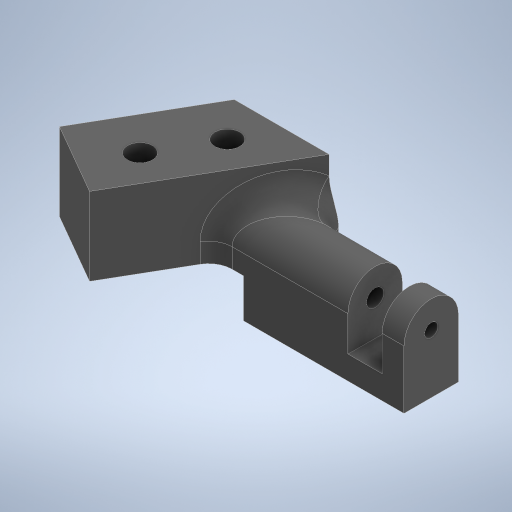
# Autodesk Inventor part: chain_base_connector
Saved by Autodesk Inventor 2024.1 (Build 281209000, 209)
## iProperties
Created: 2025-01-18
Part Number: chain_base_connector
Material: 一般
Document SubType Name: Modeling
Designer: hibik
Density: 1 g/cm^3
Appearance: 既定
Author: hibik
Autodesk Inventor part; units mm, degrees
ref_plane "YZ Plane" through (0, 0, 0) normal (1, 0, 0) x (0, 1, 0)
ref_plane "XZ Plane" through (0, 0, 0) normal (0, 1, 0) x (-1, 0, 0)
ref_plane "XY Plane" through (0, 0, 0) normal (0, 0, 1) x (1, 0, 0)
sketch "スケッチ1" plane through (0, 0, 0) normal (0, 1, 0) x (-1, 0, 0)
  line L0 (0, 0) -> (0, -18) construction
  line L1 (10, 0) -> (10, -23.7735) construction
  line L2 (10, -23.7735) -> (1.7863, -38)
  line L3 (10, -23.7735) -> (0, -18)
  line L4 (1.7863, -38) -> (-11.547, -38)
  line L5 (0, -18) -> (-11.547, -38) construction
  line L6 (-10.3923, -38) -> (0.866, -18.5)
  line L7 (9.5, -24.6395) -> (-0.9082, -18.6303)
  line L8 (-19, -38) -> (-29, -38)
  line L9 (-29, -38) -> (-29, 0)
  line L10 (-29, 0) -> (-19, 0)
  line L11 (-19, 0) -> (-19, -38)
  line L12 (-30, -38) -> (-30, 0.0797)
  line L13 (-5.1962, -36) -> (-29, -36)
  line L14 (-29, -36) -> (-29, -29)
  line L15 (-29, -29) -> (-5.1962, -29)
  line L16 (-5.1962, -29) -> (-5.1962, -36)
  point P0 (0.366, -19.366)
  point P1 (-9.2376, -36)
  dimension "d0" = 18
  dimension "d1" = 10
  dimension "d2" = 60
  dimension "d3" = 38
  dimension "d4" = 1
  dimension "d5" = 1
  dimension "d8" = 40
  dimension "d9" = 1
  dimension "d10" = 10
  dimension "d11" = 2
  dimension "d12" = 7
  constraints: 34 end point, 6 point on line, 5 parallel, 5 perpendicular, 3 horizontal, 3 vertical, 2 collinear
  measures "d0" distance of L0.start L0.end
  measures "d1" distance between parallel lines of L1 L0
  measures "d2" angle of L0 L3
  measures "d3" distance from line of L0.start L4
  measures "d4" distance between parallel lines of L5 L6
  measures "d5" distance between parallel lines of L3 L7
  measures "d8" distance from line of L1.start L12
  measures "d9" distance between parallel lines of L12 L9
  measures "d10" distance of L8.start L8.end
  measures "d11" distance between parallel lines of L8 L13
  measures "d12" distance of L15.end L13.start
extrude "押し出し1" add sketch "スケッチ1" along normal blind 3 contours L2 L7 L6 L3 | L2 L4 L6 L13 L16 L7 | L16 L13 L6 | L6 L13 L11 L15 | L11 L13 L9 L15
extrude "押し出し2" add sketch "スケッチ1" along normal blind 15 contours L2 L7 L6 L3 | L2 L4 L6 L13 L16 L7 | L16 L13 L6
sketch "スケッチ2" plane through (29, 0, -29) normal (1, 0, 0) x (0, 0, -1)
  circle A0 centre (3.5, 7.5) radius 0.85
  circle A1 centre (3.5, 7.5) radius 3.5
  line L0 (0, 7.5) -> (7, 7.5)
  line L1 (7, 7.5) -> (7, 3)
  line L2 (7, 3) -> (0, 3)
  line L3 (0, 3) -> (0, 7.5)
  line L4 (0, 3) -> (7, 3) projected
  line L5 (0, 0) -> (0, 3) projected
  point P0 (-29, 0)
  dimension "d16" = 7
  dimension "d15" = 1.7
  dimension "d17" = 4.5
  constraints: 8 end point, 2 collinear, 2 parallel, 2 vertical, 1 centre point, 1 coincident, 1 horizontal, 1 perpendicular, 3 other
  measures "d15" diameter of A0
  measures "d17" distance between parallel lines of L0 L2
extrude "押し出し3" add sketch "スケッチ2" against normal blind 2.8 contours L0 A1 A0 | A0 L0 A1 | L1 L2 L3 A1
ref_plane "作業平面1" through (24, 0, -29) normal (1, 0, 0) x (0, 0, -1)
mirror "ミラー1" about plane through (24, 0, -29) normal (1, 0, 0) of "押し出し3"
sketch "スケッチ3" plane through (19, 3, -29) normal (-1, 0, 0) x (0, 0, 1)
  circle A0 centre (-3.5, 4.5) radius 0.85 projected
  circle A1 centre (-3.5, 4.5) radius 1.1
  point P0 (29, -3)
  dimension "d21" = 2.2
  constraints: 1 centre point, 1 coincident
  measures "d21" diameter of A1
extrude "押し出し4" cut sketch "スケッチ3" against normal up to surface (2.8 mm away) contours A0 | A1
sketch "スケッチ5" plane through (0, 0, 0) normal (0, -1, 0) x (1, 0, 0)
  line L0 (3.814, -30.3) -> (5.4594, -33.15)
  line L1 (5.4594, -33.15) -> (3.814, -36)
  line L2 (3.814, -36) -> (0.5231, -36)
  line L3 (0.5231, -36) -> (-1.1224, -33.15)
  line L4 (-1.1224, -33.15) -> (0.5231, -30.3)
  line L5 (0.5231, -30.3) -> (3.814, -30.3)
  line L6 (-5.2246, -26.0447) -> (-3.5792, -23.1947)
  line L7 (-3.5792, -23.1947) -> (-0.2883, -23.1947)
  line L8 (-0.2883, -23.1947) -> (1.3571, -26.0447)
  line L9 (1.3571, -26.0447) -> (-0.2883, -28.8947)
  line L10 (-0.2883, -28.8947) -> (-3.5792, -28.8947)
  line L11 (-3.5792, -28.8947) -> (-5.2246, -26.0447)
  line L12 (-1.7863, -38) -> (-10, -23.7735) projected
  line L13 (10.3923, -38) -> (-1.7863, -38) projected
  circle A0 centre (2.1685, -33.15) radius 1.6
  circle A1 centre (-1.9338, -26.0447) radius 1.6
  line L14 (-10, -23.7735) -> (-0.866, -18.5) projected
  point P0 (0, 0)
  dimension "d27" = 5.7
  dimension "d28" = 3
  dimension "d29" = 2
  dimension "d31" = 3.2
  dimension "d32" = 3.2
  dimension "d58" = 6
  constraints: 24 end point, 2 centre point, 2 coincident, 2 parallel, 1 collinear, 26 other
  measures "d27" distance between parallel lines of L7 L10
  measures "d28" distance between parallel lines of L12 L11
  measures "d29" distance between parallel lines of L13 L2
  measures "d31" diameter of A0
  measures "d32" diameter of A1
  measures "d58" distance from line of L14 A1.centre
extrude "押し出し6" cut sketch "スケッチ5" against normal blind 11 contours L0 L1 L2 L3 L4 L5 | L6 L7 L8 L9 L10 L11 | A0 | A1
extrude "押し出し7" cut sketch "スケッチ5" against normal through all contours A0 | A1
sketch "スケッチ7" plane through (0, 0, 0) normal (0, -1, 0) x (1, 0, 0)
  line L0 (10.3923, -38) -> (-1.7863, -38) projected
  line L1 (8.3923, -38) -> (8.3923, -29)
  line L2 (5.1962, -29) -> (29, -29) projected
  line L3 (1.3571, -26.0447) -> (-0.2883, -28.8947) projected
  line L4 (-0.2883, -28.8947) -> (-3.5792, -28.8947) projected
  line L5 (-3.5792, -28.8947) -> (-5.2246, -26.0447) projected
  line L6 (-5.2246, -26.0447) -> (-3.5792, -23.1947) projected
  line L7 (-3.5792, -23.1947) -> (-0.2883, -23.1947) projected
  line L8 (-0.2883, -23.1947) -> (1.3571, -26.0447) projected
  line L9 (0.5231, -36) -> (-1.1224, -33.15) projected
  line L10 (-1.1224, -33.15) -> (0.5231, -30.3) projected
  line L11 (0.5231, -30.3) -> (3.814, -30.3) projected
  line L12 (3.814, -30.3) -> (5.4594, -33.15) projected
  line L13 (5.4594, -33.15) -> (3.814, -36) projected
  line L14 (3.814, -36) -> (0.5231, -36) projected
  line L15 (29, -36) -> (9.2376, -36) projected
  line L16 (29, -29) -> (29, -36) projected
  line L17 (5.1962, -29) -> (29, -29) projected
  line L18 (-0.866, -18.5) -> (5.1962, -29) projected
  line L19 (-1.7863, -38) -> (-10, -23.7735) projected
  line L20 (10.3923, -38) -> (-1.7863, -38) projected
  line L21 (9.2376, -36) -> (10.3923, -38) projected
  line L22 (-10, -23.7735) -> (-0.866, -18.5) projected
  point P0 (0, 0)
  point P1 (-1.7863, -38)
  dimension "d41" = 2
  constraints: 2 end point, 2 point on line, 1 vertical
  measures "d41" distance from line of L0.start L1
extrude "押し出し11" cut sketch "スケッチ7" against normal blind 5 contours L0 L19 L22 L18 L2 L1 | L3 L4 L5 L6 L7 L8 | L9 L10 L11 L12 L13 L14
sketch "スケッチ11" plane through (19, 3, -29) normal (-1, 0, 0) x (0, 0, 1)
  circle A0 centre (-3.5, 4.5) radius 1.1 projected
  line L0 (0, 4.5) -> (0, 0) projected
  arc A1 (0, 4.5) -> (-7, 4.5) centre (-3.5, 4.5) ccw projected
  line L1 (-7, 0) -> (-7, 4.5) projected
  line L2 (0, 0) -> (-7, 0) projected
  point P0 (29, -3)
extrude "押し出し15" add sketch "スケッチ11" along normal up to surface surface through (-0.866, 0, -18.5) normal (0.8660254, 0, 0.5)
sketch "スケッチ12" plane through (5.1962, 3, -29) normal (0, -1, 0) x (1, 0, 0)
  line L0 (3.1962, -5.5359) -> (3.1962, 0) projected
  line L1 (3.1962, 0) -> (0, 0) projected
  line L2 (3.1962, -5.5359) -> (0, 0) projected
  point P0 (-5.1962, 29)
extrude "押し出し16" cut sketch "スケッチ12" against normal up to surface (2 mm away)
fillet "フィレット4" radius 3 3 edges at (7.2169, 11, -32.5) (9.2376, 3.75, -36) (5.1962, 6.25, -29)
